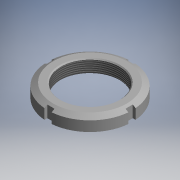
# Autodesk Inventor part: JLNSK50nut
Saved by Autodesk Inventor 2017.3 (Build 213256000, 256)
## iProperties
Part Number: JLNSK50nut
Material: Generic
Catalog Web Link: www.cadenas.de
Description: JLNK, JLNSK, JLN, JLNS_nut-Nuts for Bearings, Tooth Lock Washers for Bearings
Vendor: MISUMI
Document SubType Name: Modeling
Designer: partserver
Manufacturer: MISUMI
Mass: 20.2457 g
Surface Area: 76.1969 cm^2
Volume: 20.2457 cm^3
Density: 1 g/cm^3
Appearance: PSOLRGB-192-192-192
Category: PARTsolutions
Company: MISUMI
Title: JLNSK50nut
Author: Cadenas PARTsolutions
Comments: Nuts for Bearings, Tooth Lock Washers for Bearings
PSOL_IDENT_0: {$CADENAS_DATA\23d-libs\misumi\metric\12_bearing_holders\jlnk_nut.prj},188 {VTYP=3D},{NB=JLNSK50nut}
PSOL_IDENT_1: ,{LINA=JLNSK50nut},{NN=JLNK, JLNSK, JLN, JLNS_nut},{DATE=25.04.2017 02:57:38},{GEOMDATE=21.10.2008 1
PSOL_IDENT_2: 5:29:00},{VERSION=},{LINEID=110},{WBVAR=TS,MATN},{WBNUMERIC=}  {NB=JLNSK50nut},{LINA=JLNSK50nut},{KT=
PSOL_IDENT_3: DUMMY},{PN=JLNSK50},{NO=50},{TS=2},{TYPE=JLNSK},{MATN=SUS304},{MATNALG='1018','1018 Carbon Steel','S
PSOL_IDENT_4: US304','304 Stainless Steel'},{M=50 x 1.5},{M1=50},{PITCH=1.500},{D1=70},{D2=61},{B=11},{DD=65},{S=6
PSOL_IDENT_5: },{T=2.5},{RWS=161.5},{RWN=0.0}
NB: JLNSK50nut
NN: JLNK, JLNSK, JLN, JLNS_nut
NT: Nuts for Bearings, Tooth Lock Washers for Bearings
NBSYN: $PN.nut
LINA: JLNSK50nut
CATALOG: Misumi
PN: JLNSK50
NO: 50
TS: Set
MATN: 304 Stainless Steel
M: 50 x 1.5
M1: 50
PITCH: 1.5
D1: 70
D2: 61
B: 11
DD: 65
S: 6
T: 2.5
RWS: 161.5
RWN: 0
SUPPLIER: MISUMI
ARTICLENO: JLNSK50nut
BOMINFO: JLNSK50nut
CREATOR: CADENAS GmbH
Autodesk Inventor part; units mm, degrees
sketch "Sketch_1" plane through (0, 0, 0) normal (1, 0, 0) x (0, 1, 0)
  line L0 (0, -11) -> (0, 0)
  line L1 (25, 0) -> (24.188, -0.812)
  line L2 (24.188, -0.812) -> (24.188, -10.188)
  line L3 (24.188, -10.188) -> (25, -11)
  line L4 (25, -11) -> (30.5, -11)
  line L5 (30.5, -11) -> (35, -8.4019)
  line L6 (35, -8.4019) -> (35, 0)
  line L7 (35, 0) -> (25, 0)
  constraints: 16 end point
revolve "Revolution1" add sketch "Sketch_1" angle 360 about axis through (0, 0, -11) along (0, 0, -1)
thread "Thread1" size "M50x1.5" class "6H" standard "ISO Metric profile" full length
sketch "Sketch_2" plane through (0, 0, 0) normal (0, 0, 1) x (1, 0, 0)
  circle A0 centre (0, 0) radius 70
  arc A1 (-53.7625, -3) -> (-3, -53.7625) centre (0, 0) ccw
  line L0 (-3, -53.7625) -> (-3, -32.5)
  line L1 (-3, -32.5) -> (3, -32.5)
  line L2 (3, -32.5) -> (3, -53.7625)
  arc A2 (3, -53.7625) -> (53.7625, -3) centre (0, 0) ccw
  line L3 (53.7625, -3) -> (32.5, -3)
  line L4 (32.5, -3) -> (32.5, 3)
  line L5 (32.5, 3) -> (53.7625, 3)
  arc A3 (53.7625, 3) -> (3, 53.7625) centre (0, 0) ccw
  line L6 (3, 53.7625) -> (3, 32.5)
  line L7 (3, 32.5) -> (-3, 32.5)
  line L8 (-3, 32.5) -> (-3, 53.7625)
  arc A4 (-3, 53.7625) -> (-53.7625, 3) centre (0, 0) ccw
  line L9 (-53.7625, 3) -> (-32.5, 3)
  line L10 (-32.5, 3) -> (-32.5, -3)
  line L11 (-32.5, -3) -> (-53.7625, -3)
  constraints: 24 end point, 8 point on circle, 5 centre point
extrude "Extrusion1" cut sketch "Sketch_2" against normal blind 11
ref_plane "wash_to_nut_XY" through (0, 0, -11) normal (0, 0, 1) x (1, 0, 0)
ref_plane "wash_to_nut_YZ" through (0, 0, -11) normal (1, 0, 0) x (0, 1, 0)
ref_plane "wash_to_nut_ZX" through (0, 0, -11) normal (0, 1, 0) x (0, 0, 1)
body "Solid1"
